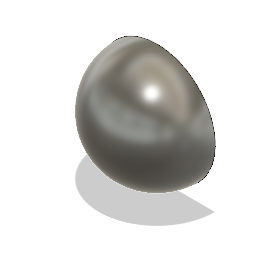
Bowl (Autodesk Fusion 360 design; units mm, degrees)
Autodesk Fusion 360 part; units mm, degrees
sketch "Sketch1" plane through (0, 0, 0) normal (0, 0, 1) x (1, 0, 0)
  arc A0 (0, -25) -> (0, 25) centre (0, 0) ccw
  arc A1 (0, -18.7312) -> (0, 18.7312) centre (0, 0) ccw
  line L0 (0, 25) -> (0, 18.7312)
  line L1 (0, -18.7312) -> (0, -25)
revolve "Revolve1" add sketch "Sketch1" angle 180 about axis through (0, 1.75, 0) along (0, -1, 0)
